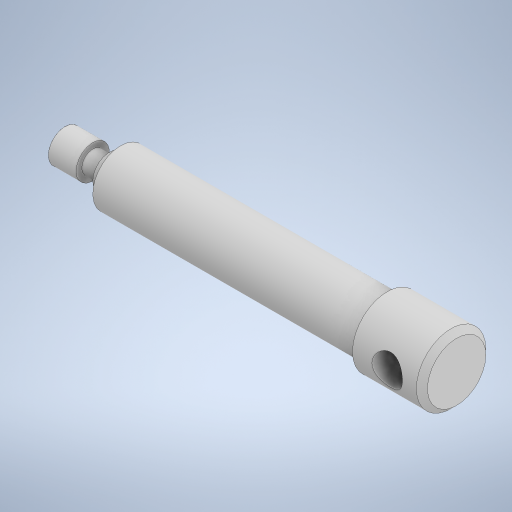
# Autodesk Inventor part: Vis de manoeuvre
Saved by Autodesk Inventor 2023.2 (Build 272271030, 271C)
## iProperties
Created: 2023-03-02
Part Number: Vis de manoeuvre
Material: Generic
Document SubType Name: Modeling
Designer: Luis Valente
Density: 1 g/cm^3
Appearance: Default
Author: Luis Valente
Autodesk Inventor part; units mm, degrees
sketch "Sketch1" plane through (0, 0, 0) normal (0, 0, 1) x (1, 0, 0)
  line L0 (0, 0) -> (121, 0)
  line L1 (121, 0) -> (121, 10)
  line L2 (121, 10) -> (0, 10)
  line L3 (0, 10) -> (0, 0)
  dimension "d0" = 121
  dimension "d1" = 10
  constraints: 8 end point, 2 parallel, 1 horizontal, 1 perpendicular
  measures "d0" distance of L2.end L1.end
  measures "d1" distance of L1.end L0.end
revolve "Revolution1" add sketch "Sketch1" angle 360 about axis through (0, 0, 0) along (1, 0, 0)
ref_plane "Work Plane1" through (60.5, 0, 0) normal (1, 0, 0) x (0, 0, -1)
sketch "Sketch3" plane through (121, 0, 0) normal (1, 0, 0) x (0, 0, -1)
  circle A0 centre (0, 0) radius 12.5
  dimension "d5" = 25
  constraints: 1 centre point, 1 coincident
  measures "d5" diameter of A0
extrude "Extrusion1" add sketch "Sketch3" against normal blind 25
chamfer "Chamfer1" distance 2 angle 45 1 edges at (121, 0, 12.5) measured on face at (121, 0, 12)
ref_plane "Work Plane2" through (121, 0, 0) normal (1, 0, 0) x (0, 0, -1)
ref_plane "Work Plane3" through (121, 0, 85.0241) normal (0, 0, 1) x (1, 0, 0)
sketch "Sketch7" plane through (121, 0, 85.0241) normal (0, 0, 1) x (1, 0, 0)
  line L0 (0, 0) -> (0, 12.2584) projected
  line L1 (0, 0) -> (-12.5, 0)
  line L2 (0, 0) -> (-25, 0) projected
  circle A0 centre (-12.5, 0) radius 5.5
  point P0 (-121, 0)
  dimension "d14" = 12.5
  dimension "d15" = 11
  constraints: 2 end point, 1 centre point, 1 coincident, 1 midpoint
  measures "d14" distance of L0.start L1.end
  measures "d15" diameter of A0
extrude "Extrusion3" cut sketch "Sketch7" against normal blind 200
sketch "Sketch8" plane through (0, 0, 0) normal (-1, 0, 0) x (0, 0, 1)
  circle A0 centre (0, 0) radius 6
  dimension "d18" = 12
  constraints: 1 centre point, 1 coincident
  measures "d18" diameter of A0
extrude "Extrusion4" add sketch "Sketch8" along normal blind 4
sketch "Sketch9" plane through (-4, 0, 0) normal (-1, 0, 0) x (0, 0, 1)
  circle A0 centre (0, 0) radius 4
  dimension "d21" = 8
  constraints: 1 centre point, 1 coincident
  measures "d21" diameter of A0
extrude "Extrusion5" add sketch "Sketch9" along normal blind 6
sketch "Sketch10" plane through (-10, 0, 0) normal (-1, 0, 0) x (0, 0, 1)
  circle A0 centre (0, 0) radius 6
  dimension "d24" = 12
  constraints: 1 centre point, 1 coincident
  measures "d24" diameter of A0
extrude "Extrusion6" add sketch "Sketch10" along normal blind 10
ref_plane "Work Plane4" through (-20, 0, 0) normal (-1, 0, 0) x (0, 0, 1)
ref_plane "Work Plane5" through (-10, 0, 0) normal (1, 0, 0) x (0, 0, -1)
sketch "Sketch18" plane through (0, 0, 0) normal (0, 1, 0) x (-1, 0, 0)
  line L0 (20, -6) -> (20, 6) projected
  line L1 (20, -6) -> (23.4641, 0)
  line L2 (20, -6) -> (26.9282, -6) construction
  line L3 (23.4641, 0) -> (20, 5.9656)
  line L4 (20, 0) -> (23.4641, 0)
  point P0 (0, 0)
  dimension "d36" = 60
  constraints: 8 end point, 2 horizontal, 1 equal length, 1 midpoint
  measures "d36" angle of L2 L1
revolve "Revolution3" add sketch "Sketch18" angle 360 about axis through (-20, 0, 0) along (-1, 0, 0) contours L0 L3 L4
body "Solid1"
